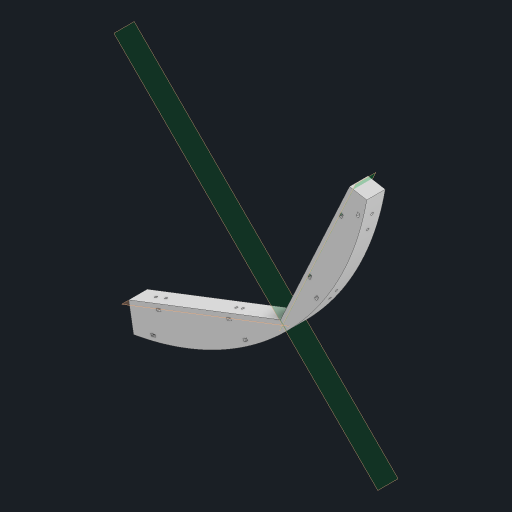
# Autodesk Inventor part: CURVA_SUPERIOR_IMPR
Saved by Autodesk Inventor 2024.3 (Build 283343000, 343)
## iProperties
Created: 2024-06-24
Part Number: CURVA_SUPERIOR_IMPR
Material: Generic
Document SubType Name: Modeling
Designer: Niler
Density: 1 g/cm^3
Appearance: Default
Author: Niler
Autodesk Inventor part; units mm, degrees
ref_plane "YZ Plane" through (0, 0, 0) normal (1, 0, 0) x (0, 1, 0)
sketch "Sketch1" plane through (0, 0, 0) normal (0, 0, 1) x (1, 0, 0)
  line L0 (-350, -350) -> (0, 0) projected
  line L1 (0, 0) -> (-35.921, 0) projected
  line L2 (-360.521, -324.6) -> (-35.921, 0) projected
  line L3 (-360.521, -324.6) -> (-350, -350) projected
  line L4 (-350, -350) -> (0, 0) projected
  line L5 (-350, -350) -> (-360.521, -324.6) projected
  line L6 (-374.6, -324.6) -> (-360.521, -324.6) projected
  line L7 (-374.6, -350) -> (-374.6, -324.6) projected
  line L8 (-374.6, -350) -> (-350, -350) projected
  line L9 (-381.5, -381.5) -> (-403.4841, -381.5)
  arc A0 (-381.5, -381.5) -> (0, 0) centre (-381.5, 0) ccw
  line L10 (0, 300) -> (-25.4, 300) projected
  line L11 (-25.4, 0) -> (-25.4, 300) projected
  line L12 (0, 0) -> (-25.4, 0) projected
  line L13 (0, 0) -> (0, 300) projected
  line L14 (-350, -350) -> (-381.5, -381.5)
  line L15 (-111.7388, -269.7612) -> (-381.5, 0)
  line L16 (-381.5, -381.5) -> (-381.5, 0)
  line L17 (-381.5, 0) -> (-5.7958, -66.2468)
  line L18 (-381.5, 0) -> (0, 0)
  line L19 (-381.5, 0) -> (-315.2532, -375.7042)
  point P0 (-324.3146, -324.3146)
  point P1 (-57.1854, -57.1854)
  dimension "d9" = 31.5
  dimension "d10" = 10
  constraints: 14 end point, 4 point on circle, 2 horizontal, 2 tangent, 1 centre point, 1 symmetric about line, 1 vertical
  measures "d9" distance between parallel lines of L9 L8
  measures "d10" angle of L18 L17
extrude "Extrusion1" add sketch "Sketch1" against normal blind 24.5 contours L0 L15 A0 L19 | L0 L17 A0 L15
ref_plane "Work Plane1" through (-381.5, 0, -24.5) normal (-0.7071068, -0.7071068, 0) x (0, 0, 1)
sketch "Sketch4" plane through (0, 0, 0) normal (0, 0, 1) x (1, 0, 0)
  arc A0 (-315.2532, -375.7042) -> (-5.7958, -66.2468) centre (-381.5, 0) ccw projected
  line L0 (-5.7958, -66.2468) -> (-57.1854, -57.1854) projected
  line L1 (-57.1854, -57.1854) -> (-324.3146, -324.3146) projected
  line L2 (-324.3146, -324.3146) -> (-315.2532, -375.7042) projected
  line L3 (0, 0) -> (-35.921, 0) projected
  line L4 (-360.521, -324.6) -> (-35.921, 0) projected
  line L5 (-360.521, -324.6) -> (-350, -350) projected
  line L6 (-350, -350) -> (0, 0) projected
  line L7 (0, 0) -> (-120.224, -261.276)
  line L8 (-120.224, -261.276) -> (-350, -350)
  line L9 (127.8879, -509.3879) -> (-466.398, 84.898) projected
  arc A1 (-315.2532, -375.7042) -> (-5.7958, -66.2468) centre (-381.5, 0) ccw projected
  point P0 (0, 0)
  point P1 (-111.7388, -269.7612)
  point P2 (-28.6302, -62.2205)
  point P3 (-321.7116, -339.0769)
  dimension "d11" = 12
  constraints: 4 end point, 1 point on circle, 1 point on line
  measures "d11" distance of point (-111.739, -269.761) L7.end
extrude "Extrusion4" cut sketch "Sketch4" against normal through all contours L2 L1 L9 L8 | L9 L1 L0 L7
sketch "Sketch8" plane through (-120.224, -261.276, -24.5) normal (-0.9084415, 0.4180121, 0) x (0, 0, 1)
  line L0 (0, 0) -> (0, 219.1176) projected
  line L1 (24.5, 0) -> (0, 0) projected
  line L2 (24.5, 219.1176) -> (24.5, 0) projected
  line L3 (0, 219.1176) -> (24.5, 219.1176) projected
  circle A0 centre (12.25, 179.1176) radius 1.65
  circle A1 centre (12.25, 79.1176) radius 1.65
  line L4 (0, 219.1176) -> (24.5, 219.1176) projected
  point P0 (24.5, 287.609)
  point P1 (12.25, 219.1176)
  dimension "d22" = 3.3
  dimension "d23" = 3.3
  dimension "d24" = 40
  dimension "d25" = 100
  constraints: 2 centre point, 2 vertical alignment, 1 midpoint
  measures "d22" diameter of A0
  measures "d23" diameter of A1
  measures "d24" distance from line of A0.centre L3
  measures "d25" distance of A1.centre A0.centre
extrude "Extrusion8" cut sketch "Sketch8" against normal through all contours A0 | A1
sketch "Sketch9" plane through (-321.7116, -339.0769, 0) normal (-0.3602119, 0.9328705, 0) x (0.9328705, 0.3602119, 0)
  line L0 (0, 24.5) -> (215.9866, 24.5) projected
  line L1 (0, 0) -> (0, 24.5) projected
  line L2 (215.9866, 0) -> (0, 0) projected
  line L3 (215.9866, 0) -> (215.9866, 24.5) projected
  circle A0 centre (40, 12.25) radius 1.65
  circle A1 centre (140, 12.25) radius 1.65
  point P0 (422.2548, 0)
  point P1 (0, 12.25)
  dimension "d28" = 100
  dimension "d29" = 40
  dimension "d30" = 3.3
  constraints: 2 centre point, 2 horizontal alignment, 1 equal radius, 1 midpoint
  measures "d28" distance of A0.centre A1.centre
  measures "d29" distance from line of A0.centre L1
  measures "d30" diameter of A0
extrude "Extrusion9" cut sketch "Sketch9" against normal through all contours A0 | A1
sketch3d "3D Sketch1"
ref_plane "Work Plane2" through (-10.9764, -90.8543, -24.5) normal (0.9712283, -0.2381502, 0) x (0.2381502, 0.9712283, 0)
sketch "Sketch11" plane through (-10.9764, -90.8543, -24.5) normal (0.9712283, -0.2381502, 0) x (0.2381502, 0.9712283, 0)
  line L0 (0, 0) -> (0, 24.5) projected
  circle A0 centre (0, 12.25) radius 1.75
  point P0 (90.8543, 24.5)
  dimension "d34" = 3.5
  constraints: 1 centre point, 1 midpoint
  measures "d34" diameter of A0
extrude "Extrusion10" cut sketch "Sketch11" against normal blind 50
ref_plane "Work Plane6" through (0, 0, -12.25) normal (0, 0, 1) x (1, 0, 0)
ref_plane "Work Plane7" through (-15.8325, -89.6636, -24.5) normal (0.9712283, -0.2381502, 0) x (0.2381502, 0.9712283, 0)
sketch "Sketch15" plane through (-15.8325, -89.6636, -24.5) normal (0.9712283, -0.2381502, 0) x (0.2381502, 0.9712283, 0)
  line L0 (-2.9, 10.5757) -> (-2.9, 13.9243)
  line L1 (-2.9, 13.9243) -> (0, 15.5986)
  line L2 (0, 15.5986) -> (2.9, 13.9243)
  line L3 (2.9, 13.9243) -> (2.9, 10.5757)
  line L4 (2.9, 10.5757) -> (0, 8.9014)
  line L5 (0, 8.9014) -> (-2.9, 10.5757)
  point P0 (90.8543, 24.5)
  point P1 (0, 12.25)
  point P2 (0, 12.25)
  dimension "d47" = 5.8
  constraints: 12 end point, 3 vertical alignment, 1 coincident, 13 other
  measures "d47" distance between parallel lines of L0 L3
extrude "Extrusion14" cut sketch "Sketch15" against normal blind 3
pattern_circular "Circular Pattern1" count 4 over 62 about axis through (-381.5, 0, 0) along (0, 0, -1) of "Extrusion14", "Extrusion10"
ref_plane "Work Plane8" through (-115.6818, -263.366, -24.5) normal (-0.9084415, 0.4180121, 0) x (0, 0, 1)
ref_plane "Work Plane9" through (-319.9105, -343.7413, 0) normal (-0.3602119, 0.9328705, 0) x (0.9328705, 0.3602119, 0)
sketch "Sketch16" plane through (-115.6818, -263.366, -24.5) normal (-0.9084415, 0.4180121, 0) x (0, 0, 1)
  circle A0 centre (12.25, 179.1176) radius 1.65 projected
  circle A1 centre (12.25, 79.1176) radius 1.65 projected
  line L0 (8.9014, 179.1176) -> (10.5757, 182.0176)
  line L1 (10.5757, 182.0176) -> (13.9243, 182.0176)
  line L2 (13.9243, 182.0176) -> (15.5986, 179.1176)
  line L3 (15.5986, 179.1176) -> (13.9243, 176.2176)
  line L4 (13.9243, 176.2176) -> (10.5757, 176.2176)
  line L5 (10.5757, 176.2176) -> (8.9014, 179.1176)
  line L6 (15.5986, 79.1176) -> (13.9243, 76.2176)
  line L7 (13.9243, 76.2176) -> (10.5757, 76.2176)
  line L8 (10.5757, 76.2176) -> (8.9014, 79.1176)
  line L9 (8.9014, 79.1176) -> (10.5757, 82.0176)
  line L10 (10.5757, 82.0176) -> (13.9243, 82.0176)
  line L11 (13.9243, 82.0176) -> (15.5986, 79.1176)
  point P0 (24.5, 287.609)
  dimension "d55" = 5.8
  dimension "d56" = 5.8
  constraints: 24 end point, 2 coincident, 2 horizontal alignment, 26 other
  measures "d55" distance between parallel lines of L4 L1
  measures "d56" distance between parallel lines of L10 L7
extrude "Extrusion15" cut sketch "Sketch16" against normal blind 3 contours A0 | A1 | L0 L1 L2 L3 L4 L5 | L6 L7 L8 L9 L10 L11
sketch "Sketch17" plane through (-319.9105, -343.7413, 0) normal (-0.3602119, 0.9328705, 0) x (0.9328705, 0.3602119, 0)
  circle A0 centre (140, 12.25) radius 1.65 projected
  circle A1 centre (40, 12.25) radius 1.65 projected
  line L0 (140, 8.9014) -> (137.1, 10.5757)
  line L1 (137.1, 10.5757) -> (137.1, 13.9243)
  line L2 (137.1, 13.9243) -> (140, 15.5986)
  line L3 (140, 15.5986) -> (142.9, 13.9243)
  line L4 (142.9, 13.9243) -> (142.9, 10.5757)
  line L5 (142.9, 10.5757) -> (140, 8.9014)
  line L6 (40, 8.9014) -> (37.1, 10.5757)
  line L7 (37.1, 10.5757) -> (37.1, 13.9243)
  line L8 (37.1, 13.9243) -> (40, 15.5986)
  line L9 (40, 15.5986) -> (42.9, 13.9243)
  line L10 (42.9, 13.9243) -> (42.9, 10.5757)
  line L11 (42.9, 10.5757) -> (40, 8.9014)
  point P0 (422.2548, 0)
  dimension "d59" = 5.8
  dimension "d60" = 5.8
  constraints: 24 end point, 2 coincident, 2 vertical alignment, 26 other
  measures "d59" distance between parallel lines of L1 L4
  measures "d60" distance between parallel lines of L7 L10
extrude "Extrusion16" cut sketch "Sketch17" against normal blind 3 contours A0 | A1 | L0 L1 L2 L3 L4 L5 | L6 L7 L8 L9 L10 L11
sketch "Sketch18" plane through (0, 0, -12.25) normal (0, 0, 1) x (1, 0, 0)
  line L0 (-16.5232, -92.4801) -> (-15.8325, -89.6636) projected
  line L1 (-15.8325, -89.6636) -> (-18.7462, -88.9491) projected
  line L2 (-18.7462, -88.9491) -> (-19.4369, -91.7657) projected
  line L3 (-16.5232, -92.4801) -> (-19.4369, -91.7657) projected
  line L4 (-15.8325, -89.6636) -> (-15.1419, -86.847) projected
  line L5 (-15.1419, -86.847) -> (-18.0556, -86.1325) projected
  line L6 (-18.0556, -86.1325) -> (-18.7462, -88.9491) projected
  line L7 (-15.8325, -89.6636) -> (-18.7462, -88.9491) projected
  line L8 (-39.5963, -98.0137) -> (-40.8085, -100.6482) projected
  line L9 (-40.8085, -100.6482) -> (-38.0832, -101.9022) projected
  line L10 (-38.0832, -101.9022) -> (-36.871, -99.2677) projected
  line L11 (-39.5963, -98.0137) -> (-36.871, -99.2677) projected
  line L12 (-40.8085, -100.6482) -> (-42.0208, -103.2827) projected
  line L13 (-42.0208, -103.2827) -> (-39.2954, -104.5367) projected
  line L14 (-39.2954, -104.5367) -> (-38.0832, -101.9022) projected
  line L15 (-40.8085, -100.6482) -> (-38.0832, -101.9022) projected
  line L16 (-82.6097, -191.4923) -> (-83.822, -194.1268) projected
  line L17 (-83.822, -194.1268) -> (-81.0966, -195.3808) projected
  line L18 (-81.0966, -195.3808) -> (-79.8844, -192.7464) projected
  line L19 (-82.6097, -191.4923) -> (-79.8844, -192.7464) projected
  line L20 (-81.3975, -188.8578) -> (-82.6097, -191.4923) projected
  line L21 (-82.6097, -191.4923) -> (-79.8844, -192.7464) projected
  line L22 (-79.8844, -192.7464) -> (-78.6722, -190.1119) projected
  line L23 (-81.3975, -188.8578) -> (-78.6722, -190.1119) projected
  line L24 (-71.0084, -212.9489) -> (-69.3682, -210.5573) projected
  line L25 (-69.3682, -210.5573) -> (-71.8422, -208.8605) projected
  line L26 (-71.8422, -208.8605) -> (-73.4825, -211.2521) projected
  line L27 (-71.0084, -212.9489) -> (-73.4825, -211.2521) projected
  line L28 (-72.6487, -215.3405) -> (-71.0084, -212.9489) projected
  line L29 (-71.0084, -212.9489) -> (-73.4825, -211.2521) projected
  line L30 (-73.4825, -211.2521) -> (-75.1227, -213.6437) projected
  line L31 (-72.6487, -215.3405) -> (-75.1227, -213.6437) projected
  line L32 (-166.1449, -308.8275) -> (-163.7661, -307.1687) projected
  line L33 (-163.7661, -307.1687) -> (-165.4821, -304.7079) projected
  line L34 (-165.4821, -304.7079) -> (-167.8609, -306.3667) projected
  line L35 (-166.1449, -308.8275) -> (-167.8609, -306.3667) projected
  line L36 (-168.5236, -310.4863) -> (-166.1449, -308.8275) projected
  line L37 (-166.1449, -308.8275) -> (-167.8609, -306.3667) projected
  line L38 (-167.8609, -306.3667) -> (-170.2396, -308.0255) projected
  line L39 (-168.5236, -310.4863) -> (-170.2396, -308.0255) projected
  line L40 (-186.6033, -292.267) -> (-189.3087, -293.3116) projected
  line L41 (-189.3087, -293.3116) -> (-188.228, -296.1102) projected
  line L42 (-188.228, -296.1102) -> (-185.5227, -295.0656) projected
  line L43 (-186.6033, -292.267) -> (-185.5227, -295.0656) projected
  line L44 (-189.3087, -293.3116) -> (-192.014, -294.3562) projected
  line L45 (-192.014, -294.3562) -> (-190.9334, -297.1548) projected
  line L46 (-190.9334, -297.1548) -> (-188.228, -296.1102) projected
  line L47 (-189.3087, -293.3116) -> (-188.228, -296.1102) projected
  line L48 (-288.9977, -364.9597) -> (-289.7348, -362.0517) projected
  line L49 (-288.9977, -364.9597) -> (-286.1866, -364.2472) projected
  line L50 (-286.1866, -364.2472) -> (-286.9237, -361.3392) projected
  line L51 (-286.9237, -361.3392) -> (-289.7348, -362.0517) projected
  line L52 (-288.9977, -364.9597) -> (-289.7348, -362.0517) projected
  line L53 (-291.8089, -365.6722) -> (-288.9977, -364.9597) projected
  line L54 (-288.9977, -364.9597) -> (-289.7348, -362.0517) projected
  line L55 (-289.7348, -362.0517) -> (-292.5459, -362.7642) projected
  line L56 (-291.8089, -365.6722) -> (-292.5459, -362.7642) projected
  line L57 (-282.5957, -329.3328) -> (-285.301, -330.3774) projected
  line L58 (-285.301, -330.3774) -> (-284.2204, -333.176) projected
  line L59 (-284.2204, -333.176) -> (-281.5151, -332.1314) projected
  line L60 (-282.5957, -329.3328) -> (-281.5151, -332.1314) projected
  line L61 (-279.8904, -328.2882) -> (-282.5957, -329.3328) projected
  line L62 (-282.5957, -329.3328) -> (-281.5151, -332.1314) projected
  line L63 (-281.5151, -332.1314) -> (-278.8098, -331.0868) projected
  line L64 (-279.8904, -328.2882) -> (-278.8098, -331.0868) projected
  point P0 (0, 0)
extrude "Extrusion17" cut sketch "Sketch18" along normal through all
sketch "Sketch5" plane through (-381.5, 0, -24.5) normal (-0.7071068, -0.7071068, 0) x (0, 0, 1)
  line L0 (-84.2203, -428.227) -> (143.9415, -428.227)
  line L1 (143.9415, -428.227) -> (143.9415, -225.904)
  line L2 (143.9415, -225.904) -> (-84.2203, -225.904)
  line L3 (-84.2203, -225.904) -> (-84.2203, -428.227)
  point P0 (24.5, -269.7612)
  constraints: 8 end point, 2 parallel, 1 horizontal, 1 perpendicular
sketch "Sketch7" plane through (-381.5, 0, -24.5) normal (-0.7071068, -0.7071068, 0) x (0.7071068, -0.7071068, 0)
  line L0 (369.5, 24.5) -> (369.5, 0) projected
  line L1 (369.5, 24.5) -> (381.5, 24.5) projected
  line L2 (381.5, 24.5) -> (381.5, 0) projected
  line L3 (381.5, 0) -> (369.5, 0) projected
  line L4 (365.6, 20.6) -> (365.6, 3.9)
  line L5 (365.6, 3.9) -> (385.4, 3.9)
  line L6 (385.4, 3.9) -> (385.4, 20.6)
  line L7 (385.4, 20.6) -> (365.6, 20.6)
  point P0 (269.7612, 24.5)
  dimension "d19" = 3.9
  constraints: 8 end point, 3 other
  measures "d19" distance between parallel lines of L1 L7
sketch "Sketch6" plane through (-381.5, 0, -24.5) normal (-0.7071068, -0.7071068, 0) x (-0.7071068, 0.7071068, 0)
  line L0 (-369.5, -24.5) -> (-369.5, -20.6) projected
  line L1 (-381.5, 0) -> (-369.5, 0) projected
  line L2 (-381.5, -24.5) -> (-381.5, -20.6) projected
  line L3 (-369.5, -24.5) -> (-381.5, -24.5) projected
  line L4 (-377.5, -4) -> (-373.5, -4)
  line L5 (-373.5, -4) -> (-373.5, -20.5)
  line L6 (-373.5, -20.5) -> (-377.5, -20.5)
  line L7 (-377.5, -20.5) -> (-377.5, -4)
  line L8 (-381.5, -3.9) -> (-369.5, -3.9) projected
  line L9 (-369.5, -20.6) -> (-381.5, -20.6) projected
  line L10 (-369.5, -3.9) -> (-369.5, 0) projected
  line L11 (-381.5, -3.9) -> (-381.5, 0) projected
  point P0 (-269.7612, -24.5)
  dimension "d16" = 4
  constraints: 8 end point, 3 other
  measures "d16" distance between parallel lines of L2 L7
body "Solid1"
